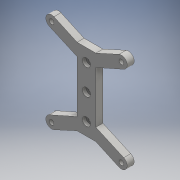
# Autodesk Inventor part: Battery Plate
Saved by Autodesk Inventor 2016 (Build 200138000, 138)
## iProperties
Created: 2017-03-22
Part Number: Battery Plate
Material: Generic
Document SubType Name: Modeling
Designer: Billy
Density: 1 g/cm^3
Appearance: Default
Author: Billy
Autodesk Inventor part; units mm, degrees
ref_plane "YZ Plane" through (0, 0, 0) normal (1, 0, 0) x (0, 1, 0)
ref_plane "XZ Plane" through (0, 0, 0) normal (0, 1, 0) x (-1, 0, 0)
ref_plane "XY Plane" through (0, 0, 0) normal (0, 0, 1) x (1, 0, 0)
sketch "Sketch1" plane through (0, 0, 0) normal (0, 1, 0) x (-1, 0, 0)
  circle A0 centre (30, -37.5) radius 2
  circle A1 centre (-30, -37.5) radius 2
  circle A2 centre (-30, 37.5) radius 2
  circle A3 centre (30, 37.5) radius 2
  arc A4 (27.9205, -42.0236) -> (32.0065, -32.9436) centre (30, -37.5) ccw
  line L0 (-8.045, -32.9204) -> (0.0364, -32.9204)
  line L1 (-8.045, -32.9204) -> (8.1178, -32.9204)
  line L2 (-8.0814, 33) -> (8.0814, 33)
  line L3 (27.9205, -42.0236) -> (8.1178, -32.9204)
  line L4 (32.0431, -32.9598) -> (8.1178, -22.3088)
  circle A5 centre (-30, -37.5) radius 2
  arc A6 (-31.9701, -32.864) -> (-27.8841, -41.944) centre (-29.9636, -37.4204) ccw
  line L5 (-27.9205, -41.9606) -> (-8.045, -32.9204)
  line L6 (-32.0067, -32.8802) -> (-8.045, -22.213)
  circle A7 centre (30, 37.5) radius 2
  circle A8 centre (-30, 37.5) radius 2
  arc A9 (32.0065, 32.9436) -> (27.9205, 42.0236) centre (30, 37.5) ccw
  line L7 (-8.0814, 33) -> (0, 33)
  line L8 (-8.0814, 33) -> (8.0814, 33)
  line L9 (27.9569, 42.0402) -> (8.0814, 33)
  line L10 (32.0278, 32.953) -> (8.1178, 22.341)
  line L11 (-27.9569, 42.0402) -> (-8.0814, 33)
  circle A10 centre (-30, 37.5) radius 2
  arc A11 (-27.9205, 42.0236) -> (-32.0065, 32.9436) centre (-30, 37.5) ccw
  line L12 (-32.0431, 32.9598) -> (-8.045, 22.2764)
  circle A12 centre (0, -22) radius 1.5
  circle A13 centre (0, 0) radius 1.5
  circle A14 centre (0, 22) radius 1.5
  line L13 (8.1178, 22.341) -> (8.1178, -22.3088)
  line L14 (-8.045, -22.213) -> (-8.045, 22.2764)
  constraints: 30 end point, 15 centre point, 12 point on circle, 8 point on line, 2 horizontal, 1 parallel
extrude "Extrusion1" add sketch "Sketch1" along normal blind 6
sketch "Sketch2" plane through (0, 6, 0) normal (0, 1, 0) x (1, 0, 0)
  circle A0 centre (-30, 37.5) radius 2 projected
  circle A1 centre (-30, 37.5) radius 3.5
  circle A2 centre (30, 37.5) radius 2 projected
  circle A3 centre (30, 37.5) radius 3.5
  circle A4 centre (-30, -37.5) radius 2 projected
  circle A5 centre (-30, -37.5) radius 3.5
  circle A6 centre (30, -37.5) radius 2 projected
  circle A7 centre (30, -37.5) radius 3.5
  point P0 (0, 0)
  dimension "d7" = 7
  dimension "d8" = 7
  dimension "d9" = 7
  dimension "d10" = 7
  constraints: 4 centre point, 4 coincident
  measures "d7" diameter of A1
  measures "d8" diameter of A3
  measures "d9" diameter of A5
  measures "d10" diameter of A7
extrude "Extrusion2" cut sketch "Sketch2" against normal blind 3 contours A1 | A3 | A5 | A6 | A7
sketch "Sketch3" plane through (0, 0, 0) normal (0, -1, 0) x (1, 0, 0)
  circle A0 centre (0, 0) radius 3.5
  circle A1 centre (0, -22) radius 1.5 projected
  circle A2 centre (0, -22) radius 3.5
  circle A3 centre (0, 22) radius 1.5 projected
  circle A4 centre (0, 22) radius 3.5
  dimension "d13" = 7
  dimension "d14" = 7
  dimension "d15" = 7
  constraints: 3 centre point, 3 coincident
  measures "d13" diameter of A0
  measures "d14" diameter of A2
  measures "d15" diameter of A4
extrude "Extrusion3" cut sketch "Sketch3" against normal blind 3
body "Solid1"
